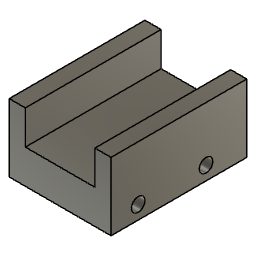
Portaservo (Autodesk Fusion 360 design; units mm, degrees)
Autodesk Fusion 360 part; units mm, degrees
note: some values were not read from the file. Set by a fixed rule: which face or edge a step refers to.
sketch "Sketch1" plane through (0, 0, 0) normal (0, 1, 0) x (1, 0, 0)
  line L0 (0, 0) -> (20.5, 0)
  line L1 (20.5, 0) -> (20.5, -10)
  line L2 (20.5, -10) -> (0, -10)
  line L3 (0, -10) -> (0, 0)
  line L4 (25.25, 0) -> (-4.75, 0)
  line L5 (-4.75, 0) -> (-4.75, -10)
  line L6 (-4.75, -10) -> (25.25, -10)
  line L7 (25.25, -10) -> (25.25, 0)
  line L8 (25.25, 0) -> (-4.75, -10) construction
  line L9 (-4.75, 0) -> (25.25, -10) construction
  line L10 (-4.75, 0) -> (-4.75, 6)
  line L11 (-4.75, 6) -> (25.25, 6)
  line L12 (25.25, 0) -> (25.25, 6)
  line L13 (-4.75, 6) -> (-4.75, 10)
  line L14 (-4.75, 10) -> (25.25, 10)
  line L15 (25.25, 10) -> (25.25, 6)
  line L16 (10.25, 0) -> (10.25, 10) construction
  line L17 (10.25, 0) -> (10.25, 2) construction
  line L18 (10.25, 2) -> (17.25, 2) construction
  line L19 (17.25, 2) -> (10.25, 2) construction
  line L20 (10.25, 2) -> (3.25, 2) construction
  circle A0 centre (3.25, 4) radius 2
  circle A1 centre (17.25, 4) radius 2
  point P0 (10.25, -5)
  dimension "d1" = 20.5
  dimension "d2" = 10
  dimension "d3" = 30
  dimension "d4" = 10
  dimension "d5" = 6
  dimension "d6" = 2
  dimension "d7" = 7
  dimension "d8" = 7
  dimension "d9" = 4
  constraint horizontal L0
  constraint vertical L1
  constraint horizontal L2
  constraint vertical L3
  constraint coincident L0.start L3.end
  constraint horizontal L4
  constraint perpendicular L4 L5
  constraint parallel L4 L6
  constraint parallel L5 L7
  constraint coincident L8 P0
  constraint coincident L9 P0
  constraint perpendicular L4 L10
  constraint perpendicular L7 L11
  constraint perpendicular L11 L12
  constraint perpendicular L11 L13
  constraint perpendicular L13 L14
  constraint perpendicular L11 L15
  constraint midpoint L4 L16.start
  constraint midpoint L14 L16.end
  constraint perpendicular L0 L17
  constraint perpendicular L16 L18
  constraint perpendicular L16 L20
  constraint coincident L20.end A0
  constraint tangent L11 A1
  constraint coincident L18.end A1
  measures "d1" distance of L0.start L0.end
  measures "d2" distance of L0.start L2.end
  measures "d3" distance of L5.end L6.end
  measures "d4" distance of L4.end L5.end
  measures "d5" distance of L4.end L10.end
  measures "d6" distance of L16.start L17.end
  measures "d7" distance of L17.end L18.end
  measures "d8" distance of L17.end L20.end
  measures "d9" diameter of A0
extrude "Extrude1" add sketch "Sketch1" along normal blind 40 contours L0 L4 L10 L11 L12 | L3 L4 L5 L6 | L1 L4 L6 L7 | L11 L13 L14 L15
sketch "Boceto3" plane through (25.25, 0, 0) normal (1, 0, 0) x (0, 1, 0)
  line L0 (0, 10) -> (0, -10)
  line L1 (0, -10) -> (40, -10)
  line L2 (40, -10) -> (40, 10)
  line L3 (40, 10) -> (0, 10)
  line L4 (0, -10) -> (0, -6)
  circle A0 centre (28, -6) radius 2
  circle A1 centre (8, -6) radius 2
  dimension "d12" = 4
  dimension "d13" = 4
  dimension "d14" = 4
  constraint coincident L0.end L1.start
  constraint perpendicular L1 L4
  measures "d12" distance of L0.end L4.end
  measures "d13" diameter of A0
  measures "d14" diameter of A1
delete_face "SuprimirCaras1" 2 faces at (5.2476, 26.6667, -3.9019) (4.4101, 26.6667, -5.6292)
delete_face "SuprimirCaras2" 1 faces at (19.2401, 13.3333, -3.8009)
hole "Agujero1" at (25.25, 8, -6) at (25.25, 28, -6) direction (-1, 0, 0) diameter 4 depth 36 tip angle 180
